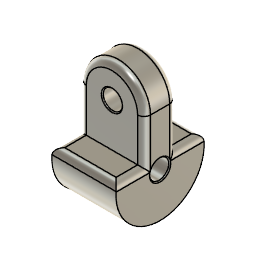
knuckle v1 (Autodesk Fusion 360 design; units mm, degrees)
Autodesk Fusion 360 part; units mm, degrees
sketch "Çizim1" plane through (0, 0, 0) normal (0, 1, 0) x (1, 0, 0)
  circle A0 centre (0, 0) radius 10
  dimension "d1" = 20
  constraint coincident A0.centre origin
  measures "d1" diameter of A0
extrude "Ekstrüzyon1" add sketch "Çizim1" along normal blind 10
sketch "Çizim2" plane through (0, 0, 0) normal (0, -1, 0) x (1, 0, 0)
  circle A0 centre (0, 0) radius 10
  line L0 (-10, 0) -> (10, 0)
  line L1 (10, 0) -> (10, -30)
  line L2 (10, -30) -> (-10, -30)
  line L3 (-10, -30) -> (-10, 0)
  dimension "d4" = 30
  constraint horizontal L0
  constraint vertical L1
  constraint horizontal L2
  constraint vertical L3
  constraint coincident A0 L0.start
  measures "d4" distance of L0.start L2.end
extrude "Ekstrüzyon2" add sketch "Çizim2" against normal blind 10 contours A0 L1 L2 L3
sketch "Çizim3" plane through (10, 0, 0) normal (1, 0, 0) x (0, 1, 0)
  line L0 (0, 0) -> (0, -30)
  line L1 (0, -30) -> (10, -30)
  line L2 (10, -30) -> (10, 0)
  line L3 (10, 0) -> (0, 0)
  circle A0 centre (5, -16.25) radius 13.75
  dimension "d7" = 27.5
  measures "d7" diameter of A0
extrude "Ekstrüzyon3" add sketch "Çizim3" against normal blind 20 contours L0 A0 | L2 A0
sketch "Çizim4" plane through (10, 0, 0) normal (1, 0, 0) x (0, 1, 0)
  line L0 (0, 0) -> (0, -3.4413)
  arc A0 (0, -3.4413) -> (0, -29.0587) centre (5, -16.25) ccw
  line L1 (0, -29.0587) -> (0, -30)
  line L2 (0, -30) -> (10, -30)
  line L3 (10, -30) -> (10, -29.0587)
  arc A1 (10, -29.0587) -> (10, -3.4413) centre (5, -16.25) ccw
  line L4 (10, -3.4413) -> (10, 0)
  line L5 (10, 0) -> (0, 0)
  circle A2 centre (5, -16.25) radius 13.75
  constraint tangent A1 A2
extrude "Ekstrüzyon4" cut sketch "Çizim4" against normal blind 35 contours L1 L2 A2 | L2 L3 A2
sketch "Çizim5" plane through (0, 0, 0) normal (0, -1, 0) x (1, 0, 0)
  line L0 (-10, -3.4413) -> (10, -3.4413)
  line L1 (10, -3.4413) -> (10, 0)
  arc A0 (10, 0) -> (-10, 0) centre (0, 0) ccw
  line L2 (-10, 0) -> (-10, -3.4413)
  circle A1 centre (0, 0) radius 3
  dimension "d12" = 6
  constraint coincident A0.centre A1.centre
  measures "d12" diameter of A1
extrude "Ekstrüzyon5" cut sketch "Çizim5" against normal blind 80 contours A1
sketch "Çizim6" plane through (10, 0, 0) normal (1, 0, 0) x (0, 1, 0)
  arc A0 (0, -3.4413) -> (10, -3.4413) centre (5, -16.25) ccw
  line L0 (10, -3.4413) -> (10, 0)
  line L1 (10, 0) -> (0, 0)
  line L2 (0, 0) -> (0, -3.4413)
  line L3 (0, -3.4413) -> (10, -3.4413)
  line L4 (10, -3.4413) -> (10, -13.4413)
  line L5 (10, -13.4413) -> (0, -13.4413)
  line L6 (0, -13.4413) -> (0, -3.4413)
  line L7 (-8.4601, -13.4413) -> (18.4601, -13.4413)
  dimension "d15" = 10
  constraint horizontal L3
  constraint vertical L4
  constraint horizontal L5
  constraint vertical L6
  constraint coincident A0.start L2.end
  constraint coincident A0 L7.start
  constraint coincident A0 L7.end
  constraint perpendicular L6 L7
  measures "d15" distance of A0.start L5.end
extrude "Ekstrüzyon6" cut sketch "Çizim6" against normal blind 39 contours A0 L6 L7 | A0 L4 L7
fillet "Radyus1" radius 2 6 edges at (0, 18.4601, -13.4413) (0, -8.4601, -13.4413) (10, -4.23, -13.4413) (10, 14.23, -13.4413) (-10, -4.23, -13.4413) (-10, 14.23, -13.4413)
fillet "Radyus2" radius 2 6 edges at (-10, 10, -7.7207) (0, 10, 10) (10, 10, -7.7207) (-10, 0, -7.7207) (0, 0, 10) (10, 0, -7.7207)
fillet "Radyus3" radius 0.3 1 edges at (-2.797, 10, -1.0848)
sketch "Çizim7" plane through (10, 0, 0) normal (1, 0, 0) x (0, 1, 0)
  line L0 (2, -15.4413) -> (-8.7262, -15.4413)
  arc A0 (-8.7262, -15.4413) -> (18.7262, -15.4413) centre (5, -16.25) ccw
  line L1 (18.7262, -15.4413) -> (8, -15.4413)
  line L2 (8, -15.4413) -> (8, 0)
  line L3 (8, 0) -> (2, 0)
  line L4 (2, 0) -> (2, -15.4413)
  circle A1 centre (5, -16.25) radius 13.75
  circle A2 centre (5, -16.25) radius 3
  dimension "d24" = 27.5
  dimension "d25" = 6
  constraint concentric A1 A2
  measures "d24" diameter of A1
  measures "d25" diameter of A2
extrude "Ekstrüzyon7" cut sketch "Çizim7" against normal blind 30 contours A2
fillet "Radyus4" radius 0.3 3 edges at (10, 2.203, -15.1652) (-10, 2.203, -17.3348) (-2.797, 0, 1.0848)
